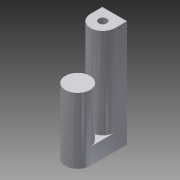
# Autodesk Inventor part: Actuator new
Saved by Autodesk Inventor 2015 (Build 190159000, 159)
## iProperties
Created: 2015-11-30
Part Number: Actuator new
Material: Aluminum 6061
Document SubType Name: Modeling
Designer: zwrouse
Density: 2.7 g/cm^3
Appearance: Aluminum - Flat
Author: zwrouse
Autodesk Inventor part; units mm, degrees
ref_plane "YZ Plane" through (0, 0, 0) normal (1, 0, 0) x (0, 1, 0)
ref_plane "XZ Plane" through (0, 0, 0) normal (0, 1, 0) x (-1, 0, 0)
ref_plane "XY Plane" through (0, 0, 0) normal (0, 0, 1) x (1, 0, 0)
sketch "Sketch1" plane through (0, 0, 0) normal (0, 1, 0) x (-1, 0, 0)
  line L0 (0, 0) -> (38.1, 0)
  line L1 (38.1, -19.05) -> (38.1, -76.2)
  line L2 (38.1, -76.2) -> (0, -76.2)
  line L3 (0, -76.2) -> (0, -19.05)
  arc A0 (38.1, -19.05) -> (0, -19.05) centre (19.05, -19.05) ccw
  dimension "d0" = 38.1
  dimension "d1" = 76.2
  constraints: 8 end point, 2 parallel, 2 point on circle, 2 tangent, 1 centre point, 1 horizontal, 1 perpendicular
  measures "d0" distance of L1.end L2.end
  measures "d1" distance of L0.end L1.end
extrude "Extrusion1" add sketch "Sketch1" along normal blind 25.4
sketch "Sketch2" plane through (0, 25.4, 0) normal (0, 1, 0) x (1, 0, 0)
  arc A0 (-38.1, 19.05) -> (0, 19.05) centre (-19.05, 19.05) ccw projected
  circle A1 centre (-19.05, 19.05) radius 19.05
  point P0 (0, 0)
  constraints: 1 centre point, 1 coincident
extrude "Extrusion2" add sketch "Sketch2" along normal blind 76.2
sketch "Sketch3" plane through (0, 25.4, 0) normal (0, 1, 0) x (1, 0, 0)
  line L0 (0, 76.2) -> (-38.1, 76.2) projected
  line L1 (0, 76.2) -> (-38.1, 76.2)
  line L2 (-38.1, 76.2) -> (-38.1, 57.8757)
  line L3 (0, 57.8757) -> (0, 76.2)
  arc A0 (-38.1, 57.8757) -> (0, 57.8757) centre (-19.05, 57.8757) ccw
  point P0 (0, 0)
  constraints: 6 end point, 2 point on circle, 1 centre point, 1 horizontal, 1 parallel, 1 perpendicular
extrude "Extrusion3" add sketch "Sketch3" along normal blind 139.7
sketch "Sketch4" plane through (0, 165.1, 0) normal (0, 1, 0) x (1, 0, 0)
  circle A0 centre (-19.05, 57.8757) radius 6.35
  arc A1 (-38.1, 57.8757) -> (0, 57.8757) centre (-19.05, 57.8757) ccw projected
  point P0 (0, 0)
  dimension "d9" = 12.7
  constraints: 1 centre point, 1 concentric
  measures "d9" diameter of A0
extrude "Extrusion4" cut sketch "Sketch4" against normal blind 121.92
body "Solid1"
